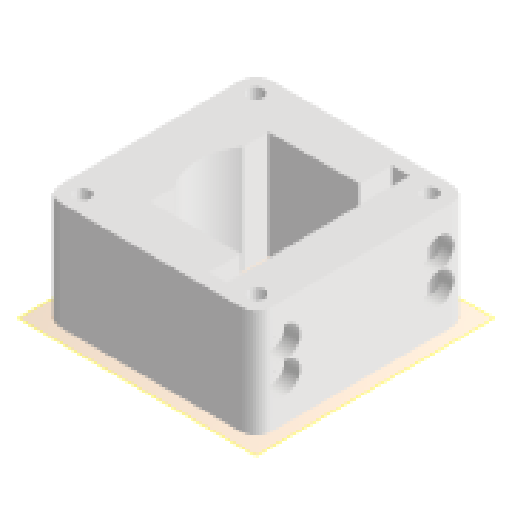
# Autodesk Inventor part: 00_Micro_Stepper_15mm_Gearbox_NEMA17Adapter
Saved by Autodesk Inventor 2024.1 (Build 281209000, 209)
## iProperties
Created: 2024-08-29
Part Number: 00_Micro_Stepper_15mm_Gearbox_NEMA17Adapter
Material: Generisch
Document SubType Name: Modeling
Designer: diederichbenedict
Density: 1 g/cm^3
Appearance: Vorgabe
Author: diederichbenedict
Autodesk Inventor part; units mm, degrees
ref_plane "YZ Plane" through (0, 0, 0) normal (1, 0, 0) x (0, 1, 0)
ref_plane "XZ Plane" through (0, 0, 0) normal (0, 1, 0) x (-1, 0, 0)
ref_plane "XY Plane" through (0, 0, 0) normal (0, 0, 1) x (1, 0, 0)
ref_plane "Arbeitsebene1" through (0, 0, 0) normal (0, 0, 1) x (1, 0, 0)
sketch "Skizze1" plane through (0, 0, 0) normal (0, 0, 1) x (1, 0, 0)
  line L0 (9.3361, 9.0616) -> (14.1886, 9.0946) projected
  line L1 (14.1529, 14.3445) -> (14.1886, 9.0946) projected
  line L2 (-14.3464, 14.1509) -> (14.1529, 14.3445) projected
  line L3 (-14.1529, -14.3445) -> (-14.3464, 14.1509) projected
  line L4 (14.3464, -14.1509) -> (-14.1529, -14.3445) projected
  line L5 (14.3108, -8.905) -> (14.3464, -14.1509) projected
  line L6 (14.3108, -8.905) -> (9.4584, -8.938) projected
  line L7 (9.4584, -8.938) -> (9.4533, -8.1804) projected
  arc A0 (9.3413, 8.3041) -> (9.4533, -8.1804) centre (0, -0.002) ccw projected
  line L8 (9.3413, 8.3041) -> (9.3361, 9.0616) projected
  circle A1 centre (-11.5623, 11.4353) radius 1.025 projected
  circle A2 centre (-11.4373, -11.5643) radius 1.025 projected
  circle A3 centre (11.5623, -11.4393) radius 1.025 projected
  circle A4 centre (11.4374, 11.5603) radius 1.025 projected
  line L9 (14.1886, 9.0946) -> (14.3108, -8.905)
  line L10 (-12, -14.002) -> (12, -14.002)
  line L11 (14, -12.002) -> (14, 11.998)
  line L12 (12, 13.998) -> (-12, 13.998)
  line L13 (-14, 11.998) -> (-14, -12.002)
  line L14 (-14, -14.002) -> (14, 13.998) construction
  line L15 (14, -14.002) -> (-14, 13.998) construction
  arc A5 (14, 11.998) -> (12, 13.998) centre (12, 11.998) ccw
  arc A6 (12, -14.002) -> (14, -12.002) centre (12, -12.002) ccw
  arc A7 (-14, -12.002) -> (-12, -14.002) centre (-12, -12.002) ccw
  arc A8 (-12, 13.998) -> (-14, 11.998) centre (-12, 11.998) ccw
  circle A9 centre (0, -0.002) radius 5
  point P0 (0, 0)
  dimension "d0" = 28
  dimension "d1" = 28
  dimension "d2" = 2
  dimension "d3" = 10
  constraints: 14 end point, 8 point on circle, 8 point on line, 8 tangent, 5 centre point, 3 equal radius, 2 midpoint, 2 parallel, 2 perpendicular, 1 coincident, 1 horizontal
  measures "d0" distance of L15.end L14.end
  measures "d1" distance of L14.end L15.start
  measures "d2" radius of A5
  measures "d3" diameter of A9
ref_plane "Arbeitsebene2" through (-46.5464, -55.86, 14.3) normal (0, 0, 1) x (1, 0, 0)
extrude "Extrusion1" add sketch "Skizze1" along normal up to surface (14.3 mm away) contours L8 A0 L7 L6 L11 A6 L10 A7 L13 A8 L12 A5 L0 | L0 L11 L6 L7 A0 L8
sketch "Skizze2" plane through (-12, 13.998, 14.3) normal (0, 0, 1) x (1, 0, 0)
  line L0 (17.9184, -1.9595) -> (17.9472, -6.2094) projected
  line L1 (18.0525, -21.7091) -> (17.9472, -6.2094) projected
  line L2 (18.0525, -21.7091) -> (18.0814, -25.959) projected
  line L3 (18.0814, -25.959) -> (20.0813, -25.9454) projected
  line L4 (19.9183, -1.9459) -> (20.0813, -25.9454) projected
  line L5 (17.9184, -1.9595) -> (19.9183, -1.9459) projected
  arc A0 (6.0307, -18.5406) -> (18.0304, -18.4591) centre (12, -14) ccw projected
  line L6 (6.0307, -18.5406) -> (6.0528, -21.7906) projected
  line L7 (6.0528, -21.7906) -> (18.0525, -21.7091) projected
  line L8 (18.0304, -18.4591) -> (18.0525, -21.7091) projected
  arc A1 (17.9693, -9.4594) -> (5.9696, -9.5409) centre (12, -14) ccw projected
  line L9 (17.9472, -6.2094) -> (17.9693, -9.4594) projected
  line L10 (5.9475, -6.2909) -> (17.9472, -6.2094) projected
  line L11 (5.9475, -6.2909) -> (5.9696, -9.5409) projected
  circle A2 centre (12, -14) radius 7.5 projected
  line L12 (17.8525, -21.7104) -> (17.8827, -26.1603)
  line L13 (17.8827, -26.1603) -> (20.2827, -26.144)
  line L14 (20.2827, -26.144) -> (20.1169, -1.7446)
  line L15 (20.1169, -1.7446) -> (17.717, -1.7609)
  line L16 (17.717, -1.7609) -> (17.7472, -6.2108)
  line L17 (18.1459, -6.0081) -> (18.1737, -10.1044)
  arc A3 (18.1737, -10.1044) -> (5.774, -10.1886) centre (12, -14) ccw
  line L18 (5.774, -10.1886) -> (5.7461, -6.0923)
  line L19 (5.7461, -6.0923) -> (18.1459, -6.0081)
  line L20 (18.2539, -21.9077) -> (5.8541, -21.9919)
  line L21 (5.8541, -21.9919) -> (5.8263, -17.8956)
  arc A4 (5.8263, -17.8956) -> (18.226, -17.8114) centre (12, -14) ccw
  line L22 (18.226, -17.8114) -> (18.2539, -21.9077)
  circle A5 centre (12, -14) radius 7.7
  point P0 (12, -13.998)
  point P1 (5.7691, -9.476)
  point P2 (5.8312, -18.6082)
  point P3 (17.8539, -21.9104)
  point P4 (17.7459, -6.0108)
  dimension "d6" = 0.2
  dimension "d7" = 0.2
  dimension "d8" = 0.2
  dimension "d9" = 0.2
  constraints: 22 end point, 4 point on circle, 3 centre point, 10 other
  measures "d6" distance between parallel lines of L4 L14
  measures "d7" distance between parallel lines of L10 L19
  measures "d8" distance between parallel lines of L7 L20
  measures "d9" radial gap between concentric circles of A2 A5
extrude "Extrusion2" cut sketch "Skizze2" against normal up to surface (14.3 mm away)
sketch "Skizze3" plane through (14, -12.002, 0) normal (1, 0, 0) x (0, 0, -1)
  ellipse E0 centre (-9.3, 22.2405) end of major axis (-8.8, 22.2405) minor radius 0.5 projected
  ellipse E1 centre (-9.3, 1.841) end of major axis (-8.8, 1.841) minor radius 0.5 projected
  ellipse E2 centre (-5.3, 22.2405) end of major axis (-4.8, 22.2405) minor radius 0.5 projected
  ellipse E3 centre (-1.3, 1.841) end of major axis (-0.8, 1.841) minor radius 0.5 projected
  ellipse E4 centre (-5.3, 1.841) end of major axis (-4.8, 1.841) minor radius 0.5 projected
  ellipse E5 centre (-1.3, 22.2405) end of major axis (-0.8, 22.2405) minor radius 0.5 projected
  line L0 (-0.8, 19.7906) -> (-14.3, 19.7906) projected
  line L1 (-14.3, 24.0405) -> (-14.3, 19.7906) projected
  line L2 (1.7, 24.0405) -> (-14.3, 24.0405) projected
  line L3 (1.7, 0.041) -> (1.7, 24.0405) projected
  line L4 (-14.3, 0.041) -> (1.7, 0.041) projected
  line L5 (-14.3, 4.2909) -> (-14.3, 0.041) projected
  line L6 (-14.3, 4.2909) -> (-0.8, 4.2909) projected
  line L7 (-0.8, 4.2909) -> (-0.8, 19.7906) projected
  point P0 (0, 12.002)
hole "Bohrung1" at (14, 10.2385, 5.3) at (14, 10.2385, 9.3) at (14, -10.161, 5.3) at (14, -10.161, 9.3) direction (-1, 0, 0) diameter 1.8 end through all counterbore diameter 4 counterbore depth 2
